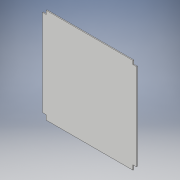
# Autodesk Inventor part: top_panel
Saved by Autodesk Inventor 2019 (Build 230136000, 136)
## iProperties
Created: 2018-07-20
Part Number: top_panel
Material: Generic
Document SubType Name: Modeling
Designer: Brian
Density: 1 g/cm^3
Appearance: Default
Author: Brian
Autodesk Inventor part; units mm, degrees
ref_plane "YZ Plane" through (0, 0, 0) normal (1, 0, 0) x (0, 1, 0)
ref_plane "XZ Plane" through (0, 0, 0) normal (0, 1, 0) x (-1, 0, 0)
ref_plane "XY Plane" through (0, 0, 0) normal (0, 0, 1) x (1, 0, 0)
sketch "Sketch1" plane through (0, 0, 0) normal (0, 0, 1) x (1, 0, 0)
  point P0 (0, 0)
sketch "Sketch2" plane through (0, 0, 0) normal (0, 0, 1) x (1, 0, 0)
  line L0 (0, 0) -> (25.4, 0)
  line L1 (25.4, 609.6) -> (0, 609.6)
  line L2 (0, 609.6) -> (0, 0)
  line L3 (635, 0.1426) -> (635, -32.8774)
  line L4 (635, -32.8774) -> (25.4, -33.02)
  line L5 (25.4, -33.02) -> (25.4, 0)
  line L6 (635, 609.7426) -> (635, 635.1426)
  line L7 (635, 635.1426) -> (25.4, 635)
  line L8 (25.4, 635) -> (25.4, 609.6)
  line L9 (635, 609.7426) -> (660.4, 609.7426)
  line L10 (660.4, 609.7426) -> (660.4, 0.1426)
  line L11 (660.4, 0.1426) -> (635, 0.1426)
  dimension "d7" = 609.6
  dimension "d8" = 609.6
  dimension "d9" = 25.4
  dimension "d10" = 25.4
  dimension "d13" = 33.02
  constraints: 24 end point, 5 parallel, 3 equal length, 3 perpendicular, 2 horizontal
  measures "d7" distance of L6.end L7.end
  measures "d8" distance of L1.end L0.start
  measures "d9" distance of L6.start L6.end
  measures "d10" distance of L10.end L3.start
  measures "d13" distance of L3.start L3.end
extrude "Extrusion1" add sketch "Sketch2" along normal blind 6.35
body "Solid1"
